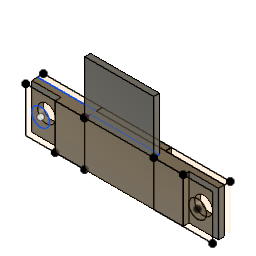
Capteur v2 (Autodesk Fusion 360 design; units mm, degrees)
Autodesk Fusion 360 part; units mm, degrees
sketch "Sketch6" plane through (0, 0, 0) normal (0, 1, 0) x (1, 0, 0)
  line L0 (0, 0) -> (-31.75, 0)
  line L1 (-31.75, 0) -> (-31.75, -7.62)
  line L2 (-31.75, -7.62) -> (0, -7.62)
  line L3 (0, -7.62) -> (0, 0)
  dimension "d16" = 7.62
  dimension "d17" = 31.75
  measures "d16" distance of L0.start
extrude "Extrude5" add sketch "Sketch6" along normal blind 3
sketch "Sketch7" plane through (0, 0, 0) normal (0, -1, 0) x (1, 0, 0)
  line L0 (0, 0) -> (0, 7.62)
  line L1 (0, 7.62) -> (-31.75, 7.62)
  line L2 (-31.75, 7.62) -> (-31.75, 0)
  line L3 (-31.75, 0) -> (0, 0)
  circle A0 centre (-29.21, 4) radius 1.5
  circle A1 centre (-2.54, 3.81) radius 1.5
  line L4 (-31.75, 7.62) -> (-26.75, 7.62)
  line L5 (-26.75, 7.62) -> (-26.75, 0)
  line L6 (-26.75, 0) -> (-31.75, 0)
  line L7 (-31.75, 0) -> (-31.75, 7.62)
  line L8 (0, 0) -> (-5, 0)
  line L9 (-5, 0) -> (-5, 7.62)
  line L10 (-5, 7.62) -> (0, 7.62)
  line L11 (0, 7.62) -> (0, 0)
  line L12 (-31.75, 7.62) -> (-21.75, 7.62)
  line L13 (-21.75, 7.62) -> (-21.75, 0)
  line L14 (-21.75, 0) -> (-31.75, 0)
  line L15 (-31.75, 0) -> (-31.75, 7.62)
  line L16 (0, 0) -> (-10, 0)
  line L17 (-10, 0) -> (-10, 7.62)
  line L18 (-10, 7.62) -> (0, 7.62)
  line L19 (0, 7.62) -> (0, 0)
  dimension "d20" = 3
  dimension "d21" = 3
  dimension "d22" = 26.67
  dimension "d24" = 2.54
  dimension "d25" = 3.81
  dimension "d30" = 5
  dimension "d31" = 5
  dimension "d36" = 10
  dimension "d37" = 10
  measures "d20" diameter of A0
  measures "d21" diameter of A1
  measures "d24" distance of L0
  measures "d25" distance of L1
  measures "d30" distance of L5 L7
  measures "d31" distance of L9 L11
  measures "d36" distance of L7 L13
  measures "d37" distance of L17 L19
extrude "Extrude8" cut sketch "Sketch7" against normal blind 1 contours L1 L2 L3 L4 L5 L6 L7 L12 L14 L15
extrude "Extrude7" cut sketch "Sketch7" against normal blind 3 contours A1
extrude "Extrude6" cut sketch "Sketch7" against normal blind 3 contours A0
extrude "Extrude9" cut sketch "Sketch7" against normal blind 1 contours L0 L1 L3 L8 L9 L10 L11 L16 L18 L19
sketch "Sketch8" plane through (0, 3, 0) normal (0, 1, 0) x (-1, 0, 0)
  circle A0 centre (29.21, 4) radius 1.5
  circle A1 centre (2.54, 3.81) radius 1.5
  line L0 (0, 7.62) -> (0, 0)
  line L1 (0, 0) -> (31.75, 0)
  line L2 (31.75, 0) -> (31.75, 7.62)
  line L3 (31.75, 7.62) -> (0, 7.62)
sketch "Sketch9" plane through (0, 0, 7.62) normal (0, 0, 1) x (-1, 0, 0)
  line L0 (5, -1) -> (0, -1)
  line L1 (0, -1) -> (0, -3)
  line L2 (0, -3) -> (31.75, -3)
  line L3 (31.75, -3) -> (31.75, -1)
  line L4 (31.75, -1) -> (26.75, -1)
  line L5 (26.75, -1) -> (26.75, 0)
  line L6 (26.75, 0) -> (5, 0)
  line L7 (5, 0) -> (5, -1)
  line L8 (31.75, -3) -> (21.75, -3)
  line L9 (21.75, -3) -> (21.75, -2)
  line L10 (21.75, -2) -> (31.75, -2)
  line L11 (31.75, -2) -> (31.75, -3)
  line L12 (0, -3) -> (10, -3)
  line L13 (10, -3) -> (10, -2)
  line L14 (10, -2) -> (0, -2)
  line L15 (0, -2) -> (0, -3)
  line L16 (21.75, -3) -> (10, -3)
  line L17 (10, -3) -> (10, -2)
  line L18 (10, -2) -> (21.75, -2)
  line L19 (21.75, -2) -> (21.75, -3)
  line L20 (21.75, 0) -> (10, 0)
  line L21 (10, 0) -> (10, -1)
  line L22 (10, -1) -> (21.75, -1)
  line L23 (21.75, -1) -> (21.75, 0)
  dimension "d39" = 10
  dimension "d40" = 1
  dimension "d45" = 11.75
  measures "d39" distance of L9 L11
  measures "d40" distance of L12 L14
extrude "Extrude12" add sketch "Sketch9" along normal blind 9 contours L6 L20 L21 L22 L23
extrude "Extrude11" cut sketch "Sketch9" against normal blind 10 contours L1 L2 L12 L13 L14 L15 L17
extrude "Extrude10" cut sketch "Sketch9" against normal blind 10 contours L2 L3 L8 L9 L10 L11 L19
